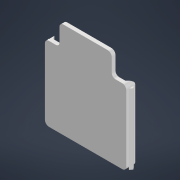
# Autodesk Inventor part: sliding cover
Saved by Autodesk Inventor 2022 (Build 260153000, 153)
## iProperties
Created: 2021-12-12
Part Number: sliding cover
Material: Generic
Document SubType Name: Modeling
Designer: nebst
Density: 1 g/cm^3
Appearance: Denim - Blue
Author: nebst
Autodesk Inventor part; units mm, degrees
ref_plane "YZ Plane" through (0, 0, 0) normal (1, 0, 0) x (0, 1, 0)
ref_plane "XZ Plane" through (0, 0, 0) normal (0, 1, 0) x (-1, 0, 0)
sketch "Sketch2" plane through (0, 0, 0) normal (0, 0, 1) x (1, 0, 0)
  line L0 (-2.676, -21.8613) -> (-2.676, 20.8107) projected
  arc A0 (-2.676, -21.8613) -> (-0.136, -24.4013) centre (-0.136, -21.8613) ccw projected
  line L1 (48.632, -24.4013) -> (-0.136, -24.4013) projected
  arc A1 (48.632, -24.4013) -> (51.172, -21.8613) centre (48.632, -21.8613) ccw projected
  line L2 (51.172, 22.3347) -> (51.172, -21.8613) projected
  arc A2 (51.172, 22.3347) -> (48.632, 24.8747) centre (48.632, 22.3347) ccw projected
  line L3 (44.06, 24.8747) -> (48.632, 24.8747) projected
  arc A3 (41.52, 27.4147) -> (44.06, 24.8747) centre (44.06, 27.4147) ccw projected
  line L4 (41.52, 36.5587) -> (41.52, 27.4147) projected
  arc A4 (41.52, 36.5587) -> (38.98, 39.0987) centre (38.98, 36.5587) ccw projected
  line L5 (9.516, 39.0987) -> (38.98, 39.0987) projected
  arc A5 (9.516, 39.0987) -> (6.976, 36.5587) centre (9.516, 36.5587) ccw projected
  line L6 (6.976, 27.4147) -> (6.976, 36.5587) projected
  arc A6 (4.436, 24.8747) -> (6.976, 27.4147) centre (4.436, 27.4147) ccw projected
  line L7 (-0.136, 24.8747) -> (4.436, 24.8747) projected
  arc A7 (-0.136, 24.8747) -> (-2.676, 22.3347) centre (-0.136, 22.3347) ccw projected
  line L8 (-2.676, 20.8107) -> (-2.676, 22.3347) projected
  arc A8 (9.516, 39.1987) -> (6.876, 36.5587) centre (9.516, 36.5587) ccw
  line L9 (9.516, 39.1987) -> (38.98, 39.1987)
  arc A9 (41.62, 36.5587) -> (38.98, 39.1987) centre (38.98, 36.5587) ccw
  line L10 (41.62, 36.5587) -> (41.62, 27.4147)
  arc A10 (41.62, 27.4147) -> (44.06, 24.9747) centre (44.06, 27.4147) ccw
  line L11 (44.06, 24.9747) -> (48.632, 24.9747)
  arc A11 (51.272, 22.3347) -> (48.632, 24.9747) centre (48.632, 22.3347) ccw
  line L12 (51.272, 22.3347) -> (51.272, -21.8613)
  arc A12 (48.632, -24.5013) -> (51.272, -21.8613) centre (48.632, -21.8613) ccw
  line L13 (48.632, -24.5013) -> (-0.136, -24.5013)
  arc A13 (-2.776, -21.8613) -> (-0.136, -24.5013) centre (-0.136, -21.8613) ccw
  line L14 (-2.776, -21.8613) -> (-2.776, 20.8107)
  line L15 (-2.776, 20.8107) -> (-2.776, 22.3347)
  arc A14 (-0.136, 24.9747) -> (-2.776, 22.3347) centre (-0.136, 22.3347) ccw
  line L16 (-0.136, 24.9747) -> (4.436, 24.9747)
  arc A15 (4.436, 24.9747) -> (6.876, 27.4147) centre (4.436, 27.4147) ccw
  line L17 (6.876, 27.4147) -> (6.876, 36.5587)
  point P0 (0, 0)
  dimension "d0" = 0.1
  constraints: 18 end point, 16 point on circle, 8 centre point, 16 other
  measures "d0" radial gap between concentric circles of A5 A8
extrude "Extrusion1" add sketch "Sketch2" against normal blind 6 contours L0 L8 A7 L7 A6 L6 A5 L5 A4 L4 A3 L3 A2 L2 A1 L1 A0 | L9 A9 L10 A10 L11 A11 L12 A12 L13 A13 L14 L15 A14 L16 A15 L17 A8
sketch "Sketch3" plane through (-0.136, -24.5013, 0) normal (0, -1, 0) x (1, 0, 0)
  line L0 (-2.69, -1.5) -> (-4.19, -3.4199) projected
  line L1 (-4.19, -3.4199) -> (-2.69, -5.3398) projected
  line L2 (-2.69, -1.5) -> (-2.64, -1.436)
  line L3 (-2.64, 0) -> (-2.64, -6) projected
  line L4 (-2.69, -5.3398) -> (-2.64, -5.4038)
  line L5 (-2.5612, -5.3423) -> (-2.6112, -5.2783)
  line L6 (-2.6112, -5.2783) -> (-4.0631, -3.4199)
  line L7 (-4.0631, -3.4199) -> (-2.6112, -1.5616)
  line L8 (-2.6112, -1.5616) -> (-2.5612, -1.4976)
  line L9 (51.408, 0) -> (51.408, -6) projected
  line L10 (51.308, -5.3398) -> (52.808, -3.4199) projected
  line L11 (52.808, -3.4199) -> (51.308, -1.5) projected
  line L12 (51.308, -1.5) -> (51.308, -5.3398) projected
  line L13 (51.408, -1.7904) -> (52.6811, -3.4199)
  line L14 (52.6811, -3.4199) -> (51.408, -5.0494)
  line L15 (51.408, -5.0494) -> (51.408, -1.7904)
  point P0 (0.136, 0)
  point P1 (-2.64, -1.5984)
  point P2 (-2.64, -5.2414)
  dimension "d5" = 0.1
  dimension "d7" = 0.1
  constraints: 18 end point, 2 point on line, 5 other
  measures "d5" distance between parallel lines of L0 L7
  measures "d7" distance between parallel lines of L11 L13
ref_plane "Work Plane1" through (-4.2928, 25.0247, -5.3398) normal (0, -1, 0) x (1, 0, 0)
extrude "Extrusion2" add sketch "Sketch3" against normal up to surface (46.836 mm away) contours L3 L6 L7 | L13 L14 L9
sketch "Sketch4" plane through (-0.136, -24.5013, 0) normal (0, -1, 0) x (1, 0, 0)
  line L0 (0.36, -2.5) -> (48.408, -2.5)
  line L1 (48.768, 0) -> (48.768, -6) projected
  line L2 (51.408, -1.7904) -> (51.408, -5.0494) projected
  line L3 (0, -6) -> (48.768, -6) projected
  line L4 (-2.64, -5.2414) -> (-2.64, -1.5984) projected
  line L5 (-2.64, 0) -> (0, 0) projected
  line L6 (-2.64, 0) -> (-2.64, -1.5984) projected
  line L7 (-2.64, -1.5984) -> (-2.64, -5.2414) projected
  line L8 (-2.64, -5.2414) -> (-2.64, -6) projected
  line L9 (0, -6) -> (-2.64, -6) projected
  line L10 (0, 0) -> (0, -6) projected
  line L11 (0, 0) -> (48.768, 0) projected
  line L12 (0, 0) -> (0, -6) projected
  line L13 (48.768, -6) -> (0, -6) projected
  line L14 (48.768, 0) -> (48.768, -6) projected
  line L15 (48.768, 0) -> (51.408, 0) projected
  line L16 (48.768, 0) -> (48.768, -6) projected
  line L17 (51.408, -6) -> (48.768, -6) projected
  line L18 (51.408, -5.0494) -> (51.408, -6) projected
  line L19 (51.408, -1.7904) -> (51.408, -5.0494) projected
  line L20 (51.408, 0) -> (51.408, -1.7904) projected
  line L21 (-2.64, -6) -> (0, -6) projected
  line L22 (-2.34, -6) -> (0.36, -2.5)
  line L23 (48.408, -2.5) -> (51.108, -6)
  line L24 (48.768, -6) -> (51.408, -6) projected
  point P0 (0.136, 0)
  point P1 (0, -2.9667)
  point P2 (48.768, -2.9667)
  dimension "d8" = 3.5
  dimension "d9" = 3
  dimension "d10" = 3
  dimension "d28" = 0.3
  dimension "d29" = 0.3
  constraints: 6 end point, 2 point on line, 1 perpendicular
  measures "d8" distance between parallel lines of L0 L3
  measures "d9" distance from line of L2 L0.end
  measures "d10" distance from line of L4 L0.start
  measures "d28" distance of L8.end L22.start
  measures "d29" distance of L17.start L23.end
extrude "Extrusion3" cut sketch "Sketch4" against normal through all contours L0 L23 L1 L3 L10 L22 | L10 L9 L22 | L23 L17 L1
sketch "Sketch5" plane through (0, 0, 0) normal (0, 0, 1) x (1, 0, 0)
  line L0 (7.174, -27.7513) -> (7.174, -25.3513) projected
  line L1 (41.322, -25.3513) -> (41.322, -27.7513) projected
  line L2 (-2.826, -21.8613) -> (-2.826, -27.9867) projected
  arc A0 (-2.826, -27.9867) -> (-0.136, -28.5513) centre (-0.136, -21.8613) ccw projected
  line L3 (-0.136, -28.5513) -> (48.632, -28.5513) projected
  arc A1 (48.632, -28.5513) -> (51.322, -27.9867) centre (48.632, -21.8613) ccw projected
  arc A2 (48.632, -24.5513) -> (51.322, -21.8613) centre (48.632, -21.8613) ccw projected
  line L4 (48.632, -24.5513) -> (-0.136, -24.5513) projected
  arc A3 (-2.826, -21.8613) -> (-0.136, -24.5513) centre (-0.136, -21.8613) ccw projected
  line L5 (-2.776, -27.9539) -> (-2.776, -21.1278)
  arc A4 (-2.776, -21.1278) -> (-0.136, -24.6013) centre (-0.136, -21.8613) ccw
  line L6 (-0.136, -24.6013) -> (48.632, -24.6013)
  arc A5 (48.632, -24.6013) -> (51.272, -22.5948) centre (48.632, -21.8613) ccw
  line L7 (51.272, -22.5948) -> (51.272, -27.9539)
  arc A6 (48.632, -28.5013) -> (51.272, -27.9539) centre (48.632, -21.8613) ccw
  line L8 (48.632, -28.5013) -> (-0.136, -28.5013)
  arc A7 (-2.776, -27.9539) -> (-0.136, -28.5013) centre (-0.136, -21.8613) ccw
  line L9 (51.272, -24.5013) -> (51.272, -21.8613) projected
  line L10 (51.272, -22.5948) -> (51.272, -21.8613)
  line L11 (38.98, 39.1987) -> (9.516, 39.1987) projected
  arc A8 (9.516, 39.1987) -> (6.876, 36.5587) centre (9.516, 36.5587) ccw projected
  line L12 (6.876, 36.5587) -> (6.876, 27.4147) projected
  arc A9 (4.436, 24.9747) -> (6.876, 27.4147) centre (4.436, 27.4147) ccw projected
  line L13 (4.436, 24.9747) -> (-0.136, 24.9747) projected
  line L14 (-0.136, -24.5013) -> (48.632, -24.5013) projected
  line L15 (48.632, 24.9747) -> (44.06, 24.9747) projected
  arc A10 (41.62, 27.4147) -> (44.06, 24.9747) centre (44.06, 27.4147) ccw projected
  line L16 (41.62, 27.4147) -> (41.62, 36.5587) projected
  arc A11 (41.62, 36.5587) -> (38.98, 39.1987) centre (38.98, 36.5587) ccw projected
  line L17 (7.174, -27.7513) -> (41.322, -27.7513) projected
  line L18 (41.322, -25.3513) -> (7.174, -25.3513) projected
  arc A12 (-0.136, 24.9747) -> (-2.776, 22.3347) centre (-0.136, 22.3347) ccw projected
  line L19 (-2.776, 22.3347) -> (-2.776, -21.8613) projected
  arc A13 (-2.776, -21.8613) -> (-0.136, -24.5013) centre (-0.136, -21.8613) ccw projected
  arc A14 (48.632, -24.5013) -> (51.272, -21.8613) centre (48.632, -21.8613) ccw projected
  line L20 (51.272, -21.8613) -> (51.272, 22.3347) projected
  arc A15 (51.272, 22.3347) -> (48.632, 24.9747) centre (48.632, 22.3347) ccw projected
  line L21 (-2.776, -21.8613) -> (-2.776, -22.5948)
  line L22 (-2.776, -24.5013) -> (-2.776, -21.8613) projected
  line L23 (51.272, -24.5013) -> (51.272, -21.8613) projected
  line L24 (51.272, -21.8613) -> (51.272, -22.5948)
  line L25 (51.322, -27.9867) -> (51.322, -21.8613) projected
  point P0 (0, 0)
  point P1 (51.322, -22.3813)
  point P2 (-2.776, -22.5948)
  dimension "d13" = 0.05
  constraints: 14 end point, 9 point on circle, 4 centre point, 1 point on line, 5 other
  measures "d13" distance between parallel lines of L2 L5
extrude "Extrusion4" add sketch "Sketch5" against normal blind 5.9 contours L0 L18 L1 L17 | L5 A13 L14 A14 L9 A2 L4 A3 | A3 L4 A2 L9 A5 L6 A4 L5 | A4 L6 A5 L7 A6 L8 A7 L5
sketch "Sketch9" plane through (-0.136, -24.5013, 0) normal (0, -1, 0) x (1, 0, 0)
  line L0 (-4.0631, -3.4199) -> (-2.64, -5.2414) projected
  line L1 (-2.64, -5.2414) -> (-2.64, -1.5984) projected
  line L2 (-2.64, -1.5984) -> (-4.0631, -3.4199) projected
  line L3 (52.6811, -3.4199) -> (51.408, -1.7904) projected
  line L4 (51.408, -1.7904) -> (51.408, -5.0494) projected
  line L5 (51.408, -5.0494) -> (52.6811, -3.4199) projected
  point P0 (0.136, 0)
extrude "Extrusion8" add sketch "Sketch9" along normal blind 10
sketch "Sketch6" plane through (0, 0, -5.9) normal (0, 0, -1) x (-1, 0, 0)
  line L0 (-47.2713, -25.8513) -> (-47.2713, -27.2513) projected
  line L1 (-41.322, -27.2513) -> (-7.174, -27.2513) projected
  line L2 (-7.174, -25.8513) -> (-41.322, -25.8513) projected
  line L3 (-1.174, -27.2513) -> (-1.174, -25.8513) projected
  line L4 (-37.2713, -26.0513) -> (-37.2713, -27.2513)
  line L5 (-37.2713, -27.2513) -> (-11.174, -27.2513)
  line L6 (-11.174, -27.2513) -> (-11.174, -26.0513)
  line L7 (-11.174, -26.0513) -> (-37.2713, -26.0513)
  point P0 (0, 0)
  dimension "d16" = 10
  dimension "d30" = 10
  dimension "d31" = 0.2
  dimension "d32" = 0
  constraints: 8 end point
  measures "d16" distance between parallel lines of L0 L4
  measures "d30" distance between parallel lines of L3 L6
  measures "d31" distance between parallel lines of L2 L7
  measures "d32" distance between parallel lines of L1 L5
extrude "Extrusion5" add sketch "Sketch6" along normal blind 0.5
chamfer "Chamfer1" distance 0.5 angle 45 2 edges at (24.2226, -26.0513, -6.4) (24.2226, -27.2513, -6.4)
sketch "Sketch7" plane through (9.516, 39.1987, 0) normal (0, 1, 0) x (1, 0, 0)
  line L0 (26.464, 1.4) -> (26.464, 2.6) projected
  line L1 (3, 1.4) -> (26.464, 1.4) projected
  line L2 (26.464, 2.6) -> (3, 2.6) projected
  line L3 (3, 2.6) -> (3, 1.4) projected
  line L4 (29.464, 2.5) -> (0, 2.5) projected
  line L5 (25.464, 2.5) -> (4, 2.5)
  line L6 (4, 2.5) -> (4, 1.5)
  line L7 (4, 1.5) -> (25.464, 1.5)
  line L8 (25.464, 1.5) -> (25.464, 2.5)
  point P0 (-9.516, 0)
  point P1 (26.364, 2.5)
  point P2 (3.1, 2.5)
  point P3 (4, 2.5)
  dimension "d22" = 1
  dimension "d23" = 0.1
  dimension "d24" = 1
  constraints: 8 end point, 2 parallel, 1 horizontal, 1 perpendicular, 2 other
  measures "d22" distance between parallel lines of L3 L6
  measures "d23" distance between parallel lines of L1 L7
  measures "d24" distance between parallel lines of L0 L8
extrude "Extrusion6" add sketch "Sketch7" along normal blind 1.5 contours L8 L7 L6 L4
sketch "Sketch8" plane through (0, 0, 0) normal (0, 0, 1) x (1, 0, 0)
  line L0 (2.224, -25.5013) -> (22.224, -25.5013) construction
  line L1 (2.224, -26.5013) -> (22.224, -26.5013)
  line L2 (22.224, -24.5013) -> (2.224, -24.5013)
  arc A0 (2.224, -24.5013) -> (2.224, -26.5013) centre (2.224, -25.5013) ccw
  arc A1 (22.224, -26.5013) -> (22.224, -24.5013) centre (22.224, -25.5013) ccw
  line L3 (38.98, 39.1987) -> (9.516, 39.1987) projected
  line L4 (-2.776, 22.3347) -> (-2.776, -27.9539) projected
  arc A2 (2.224, -20.5013) -> (2.224, -22.5013) centre (2.224, -21.5013) ccw
  line L5 (22.224, -20.5013) -> (2.224, -20.5013)
  line L6 (2.224, -22.5013) -> (22.224, -22.5013)
  arc A3 (22.224, -22.5013) -> (22.224, -20.5013) centre (22.224, -21.5013) ccw
  arc A4 (2.224, -16.5013) -> (2.224, -18.5013) centre (2.224, -17.5013) ccw
  line L7 (22.224, -16.5013) -> (2.224, -16.5013)
  line L8 (2.224, -18.5013) -> (22.224, -18.5013)
  arc A5 (22.224, -18.5013) -> (22.224, -16.5013) centre (22.224, -17.5013) ccw
  arc A6 (2.224, -12.5013) -> (2.224, -14.5013) centre (2.224, -13.5013) ccw
  line L9 (22.224, -12.5013) -> (2.224, -12.5013)
  line L10 (2.224, -14.5013) -> (22.224, -14.5013)
  arc A7 (22.224, -14.5013) -> (22.224, -12.5013) centre (22.224, -13.5013) ccw
  arc A8 (2.224, -8.5013) -> (2.224, -10.5013) centre (2.224, -9.5013) ccw
  line L11 (22.224, -8.5013) -> (2.224, -8.5013)
  line L12 (2.224, -10.5013) -> (22.224, -10.5013)
  arc A9 (22.224, -10.5013) -> (22.224, -8.5013) centre (22.224, -9.5013) ccw
  line L13 (-0.136, -28.5013) -> (48.632, -28.5013) projected
  line L14 (24.248, 22.7443) -> (24.248, 17.9951)
  line L15 (46.272, -25.5013) -> (26.272, -25.5013) construction
  line L16 (46.272, -26.5013) -> (26.272, -26.5013)
  line L17 (26.272, -24.5013) -> (46.272, -24.5013)
  arc A10 (46.272, -26.5013) -> (46.272, -24.5013) centre (46.272, -25.5013) ccw
  arc A11 (26.272, -24.5013) -> (26.272, -26.5013) centre (26.272, -25.5013) ccw
  arc A12 (46.272, -22.5013) -> (46.272, -20.5013) centre (46.272, -21.5013) ccw
  line L18 (26.272, -20.5013) -> (46.272, -20.5013)
  line L19 (46.272, -22.5013) -> (26.272, -22.5013)
  arc A13 (26.272, -20.5013) -> (26.272, -22.5013) centre (26.272, -21.5013) ccw
  arc A14 (46.272, -18.5013) -> (46.272, -16.5013) centre (46.272, -17.5013) ccw
  line L20 (26.272, -16.5013) -> (46.272, -16.5013)
  line L21 (46.272, -18.5013) -> (26.272, -18.5013)
  arc A15 (26.272, -16.5013) -> (26.272, -18.5013) centre (26.272, -17.5013) ccw
  arc A16 (46.272, -14.5013) -> (46.272, -12.5013) centre (46.272, -13.5013) ccw
  line L22 (26.272, -12.5013) -> (46.272, -12.5013)
  line L23 (46.272, -14.5013) -> (26.272, -14.5013)
  arc A17 (26.272, -12.5013) -> (26.272, -14.5013) centre (26.272, -13.5013) ccw
  arc A18 (46.272, -10.5013) -> (46.272, -8.5013) centre (46.272, -9.5013) ccw
  line L24 (26.272, -8.5013) -> (46.272, -8.5013)
  line L25 (46.272, -10.5013) -> (26.272, -10.5013)
  arc A19 (26.272, -8.5013) -> (26.272, -10.5013) centre (26.272, -9.5013) ccw
  point P0 (0, 0)
  point P1 (12.224, -25.5013)
  point P2 (36.272, -25.5013)
  dimension "d33" = 2
  dimension "d34" = 20
  dimension "d35" = 15
  dimension "d38" = 4
  dimension "d43" = 3
  dimension "d45" = 27.024
  constraints: 50 end point, 40 point on circle, 31 symmetric about line, 20 centre point, 4 tangent, 2 vertical, 1 horizontal, 1 midpoint, 1 parallel, 50 other
  measures "d33" distance between parallel lines of L2 L1
  measures "d34" distance of L0.start L0.end
  measures "d35" distance from line of L4 point (12.224, -25.501)
  measures "d38" distance of L0.start A2.centre
  measures "d43" distance between parallel lines of L13 L0
  measures "d45" distance between parallel lines of L4 L14
extrude "Extrusion7" cut sketch "Sketch8" against normal blind 1
sketch "Sketch10" plane through (0, 0, 0) normal (0, 0, 1) x (1, 0, 0)
  arc A0 (-2.826, -27.9867) -> (-0.136, -28.5513) centre (-0.136, -21.8613) ccw projected
  arc A1 (-6.826, -21.8613) -> (-2.826, -27.9867) centre (-0.136, -21.8613) ccw projected
  arc A2 (51.322, -27.9867) -> (55.322, -21.8613) centre (48.632, -21.8613) ccw projected
  arc A3 (48.632, -28.5513) -> (51.322, -27.9867) centre (48.632, -21.8613) ccw projected
  line L0 (-6.826, -21.8613) -> (-0.136, -21.8613)
  line L1 (-0.136, -21.8613) -> (-0.136, -34.9478)
  line L2 (-0.136, -34.9478) -> (-6.826, -34.9478)
  line L3 (-6.826, -34.9478) -> (-6.826, -21.8613)
  line L4 (55.322, -21.8613) -> (48.632, -21.8613)
  line L5 (48.632, -21.8613) -> (48.632, -36.8339)
  line L6 (48.632, -36.8339) -> (55.322, -36.8339)
  line L7 (55.322, -36.8339) -> (55.322, -21.8613)
  point P0 (0, 0)
  point P1 (-0.136, -28.5513)
  constraints: 16 end point, 4 parallel, 2 horizontal, 2 perpendicular
extrude "Extrusion9" cut sketch "Sketch10" against normal blind 10 contours A0 L1 L2 L3 A1 | A2 L7 L6 L5 A3
body "Solid1"
